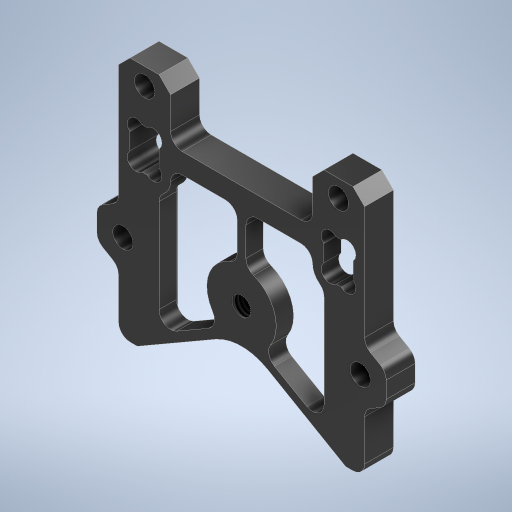
# Autodesk Inventor part: LegBaseBackFulcrumFrame
Saved by Autodesk Inventor 2024.2 (Build 282272000, 272)
## iProperties
Created: 2024-01-07
Part Number: LegBaseBackFulcrumFrame
Material: Aluminum 7075
Document SubType Name: Modeling
Designer: Masato Kubotera
Density: 2.81 g/cm^3
Appearance: Glossy - Black
Mass: 9.74355 g
Surface Area: 36.5407 cm^2
Volume: 3.46745 cm^3
Vendor: meviy
Author: Masato Kubotera
Autodesk Inventor part; units mm, degrees
ref_plane "YZ Plane" through (0, 0, 0) normal (1, 0, 0) x (0, 1, 0)
ref_plane "XZ Plane" through (0, 0, 0) normal (0, 1, 0) x (-1, 0, 0)
ref_plane "XY Plane" through (0, 0, 0) normal (0, 0, 1) x (1, 0, 0)
sketch "Sketch1" plane through (0, 0, 0) normal (1, 0, 0) x (0, 1, 0)
  line L0 (-16, 16) -> (16, 16) construction
  line L1 (16, 16) -> (16, -27) construction
  line L2 (16, -27) -> (-16, -27) construction
  line L3 (-16, -27) -> (-16, 16) construction
  line L4 (-16, 16) -> (16, -27) construction
  line L5 (16, 16) -> (-16, -27) construction
  line L6 (-13.5, 13) -> (13.5, 13) construction
  line L7 (13.5, 13) -> (13.5, -14) construction
  line L8 (13.5, -14) -> (-13.5, -14) construction
  line L9 (-13.5, -14) -> (-13.5, 13) construction
  line L10 (-13.5, 13) -> (13.5, -14) construction
  line L11 (13.5, 13) -> (-13.5, -14) construction
  line L12 (0, 18) -> (0, -27)
  circle A0 centre (0, -15) radius 8 construction
  circle A1 centre (0, 0) radius 6 construction
  line L13 (25, 27.5) -> (-25, 27.5) construction
  line L14 (19.3, 18.55) -> (14.2, 18.55)
  line L15 (14.2, 18.55) -> (14.2, 11.45)
  line L16 (14.2, 11.45) -> (19.3, 11.45)
  line L17 (19.3, 11.45) -> (19.3, 18.55)
  line L18 (19.3, 18.55) -> (14.2, 11.45) construction
  line L19 (14.2, 18.55) -> (19.3, 11.45) construction
  line L20 (-16.05, -6) -> (-16.05, 16)
  line L21 (-16.05, 16) -> (16.05, 16)
  line L22 (16.05, 16) -> (16.05, -13.8742)
  line L23 (12.25, 27.5) -> (12.25, 18)
  line L24 (12.25, 18) -> (-12.25, 18)
  line L25 (-12.25, 18) -> (-12.25, 27.5)
  arc A2 (19.3, 16.4287) -> (17.1787, 18.55) centre (18.2393, 17.4893) ccw
  line L26 (19.3, 15) -> (14.2, 15) construction
  line L27 (16.75, 18.55) -> (16.75, 11.45) construction
  arc A3 (16.3213, 18.55) -> (14.2, 16.4287) centre (15.2607, 17.4893) ccw
  arc A4 (17.1787, 11.45) -> (19.3, 13.5713) centre (18.2393, 12.5107) ccw
  arc A5 (14.2, 13.5713) -> (16.3213, 11.45) centre (15.2607, 12.5107) ccw
  line L28 (17.5, -1.7321) -> (17.5, 1.7321) construction
  line L29 (17.5, 1.7321) -> (20.5, 3.4641) construction
  line L30 (20.5, 3.4641) -> (23.5, 1.7321) construction
  line L31 (23.5, 1.7321) -> (23.5, -1.7321) construction
  line L32 (23.5, -1.7321) -> (20.5, -3.4641) construction
  line L33 (20.5, -3.4641) -> (17.5, -1.7321) construction
  line L34 (-25, 5) -> (19.25, 5) construction
  circle A6 centre (20.5, 0) radius 2.75 construction
  line L35 (16.05, 0) -> (25, 0) construction
  line L36 (20.5, 3.5218) -> (23.55, 1.7609)
  line L37 (23.55, 1.7609) -> (23.55, -1.7609)
  line L38 (23.55, -1.7609) -> (20.5, -3.5218)
  line L39 (20.5, -3.5218) -> (17.45, -1.7609)
  line L40 (17.45, -1.7609) -> (17.45, 1.7609)
  line L41 (17.45, 1.7609) -> (20.5, 3.5218)
  arc A7 (21.799, 2.7718) -> (19.201, 2.7718) centre (20.5, 2.0218) ccw
  arc A8 (18.749, 2.5109) -> (17.45, 0.2609) centre (18.749, 1.0109) ccw
  arc A9 (17.45, -0.2609) -> (18.749, -2.5109) centre (18.749, -1.0109) ccw
  arc A10 (19.201, -2.7718) -> (21.799, -2.7718) centre (20.5, -2.0218) ccw
  arc A11 (22.251, -2.5109) -> (23.55, -0.2609) centre (22.251, -1.0109) ccw
  arc A12 (23.55, 0.2609) -> (22.251, 2.5109) centre (22.251, 1.0109) ccw
  line L42 (21.25, 27.5) -> (21.25, 4.7631)
  line L43 (21.25, 4.7631) -> (25, 2.5981)
  line L44 (4.5, -7.2058) -> (18, -15)
  line L45 (21.25, -4.7631) -> (25, -2.5981)
  line L46 (21.25, -4.7631) -> (21.25, -15)
  arc A13 (4.5, -7.2058) -> (0, -6) centre (0, -15) ccw
  line L47 (19.25, 18.5) -> (14.25, 18.5) construction
  line L48 (14.25, 18.5) -> (14.25, 11.5) construction
  line L49 (14.25, 11.5) -> (19.25, 11.5) construction
  line L50 (19.25, 11.5) -> (19.25, 18.5) construction
  line L51 (19.25, 18.5) -> (14.25, 11.5) construction
  line L52 (14.25, 18.5) -> (19.25, 11.5) construction
  arc A14 (5.25, -5.9067) -> (3.2786, -5.025) centre (0, -15) ccw
  line L53 (5.25, -5.9067) -> (14.25, -11.1029)
  line L54 (14.25, -11.1029) -> (14.25, 9.686)
  line L55 (0, 0) -> (25, 0) construction
  line L56 (0.75, 14.5) -> (12.7, 14.5)
  line L57 (12.7, 14.5) -> (12.7, 14.0737)
  arc A15 (12.7, 14.0737) -> (14.25, 9.686) centre (15.2607, 12.5107) ccw
  arc A16 (3.2786, -5.025) -> (0.75, 5.9529) centre (0, 0) ccw
  line L58 (0.75, 14.5) -> (0.75, 5.9529)
  line L59 (25, 2.5981) -> (25, -2.5981)
  line L60 (21.25, 27.5) -> (12.25, 27.5)
  line L61 (18, -15) -> (21.25, -15)
  point P0 (0, -5.5)
  point P1 (0, -0.5)
  point P2 (16.05, -6)
  point P3 (16.3213, 11.45)
  point P4 (14.2, 13.5713)
  point P5 (14.2, 16.4287)
  point P6 (16.3213, 18.55)
  point P7 (19.3, 13.5713)
  point P8 (17.1787, 11.45)
  point P9 (17.45, 1.7609)
  point P10 (17.45, -1.7609)
  point P11 (20.5, -3.5218)
  point P12 (23.55, -1.7609)
  point P13 (23.55, 1.7609)
  point P14 (17.45, 0.2609)
  point P15 (17.45, -0.2609)
  point P16 (18.749, -2.5109)
  point P17 (19.201, -2.7718)
  point P18 (21.799, -2.7718)
  point P19 (22.251, -2.5109)
  point P20 (23.55, -0.2609)
  point P21 (23.55, 0.2609)
  point P22 (22.251, 2.5109)
  point P23 (18.749, 2.5109)
  point P24 (16.75, 24.5)
  point P25 (16.75, 15)
  point P26 (16.75, 15)
  point P27 (16.05, 11.2351)
  point P28 (14.2, 16)
  point P29 (0, 16)
  point P30 (5.9529, -0.75)
  dimension "d0" = 32
  dimension "d1" = 43
  dimension "d2" = 27
  dimension "d4" = 16
  dimension "d5" = 15
  dimension "d12" = 8.5
  dimension "d13" = 9.5
  dimension "d72" = 12
  dimension "d75" = 27.5
  dimension "d83" = 2
  dimension "d84" = 1.5
  dimension "d86" = 6
  dimension "d89" = 5
  dimension "d90" = 5.5
  dimension "d91" = 0.05
  dimension "d94" = 360
  dimension "d104" = 3
  dimension "d110" = 60
  dimension "d111" = 0.05
  dimension "d112" = 0.05
  dimension "d113" = 9
  dimension "d114" = 6.5
  dimension "d115" = 28.5
  dimension "d116" = 2
  dimension "d117" = 5
  dimension "d118" = 0.05
  dimension "d120" = 1.5
  dimension "d124" = 1.5
  dimension "d127" = 1.5
  dimension "d129" = 1.5
  dimension "d130" = 1.5
  dimension "d131" = 1.5
  dimension "d132" = 1.5
  dimension "d134" = 1.5
  dimension "d135" = 27
  constraints: 125 end point, 32 point on circle, 18 point on line, 17 centre point, 15 midpoint, 11 symmetric about line, 9 horizontal, 8 coincident, 8 parallel, 8 vertical, 4 collinear, 4 perpendicular, 3 tangent, 1 equal radius, 63 other
  measures "d0" distance of L1.end L2.end
  measures "d1" distance of L0.end L1.end
  measures "d2" distance of L7.end L8.end
  measures "d4" diameter of A0
  measures "d5" distance of A0.centre point (0, 0)
  measures "d12" distance from line of point (0, -5.5) L8
  measures "d13" distance of A0.centre point (0, -5.5)
  measures "d72" diameter of A1
  measures "d75" distance from line of L13 point (0, 0)
  measures "d83" distance between parallel lines of L21 L24
  measures "d84" radius of A2
  measures "d86" distance between parallel lines of L28 L31
  measures "d89" distance from line of point (0, 0) L34
  measures "d90" diameter of A6
  measures "d91" distance between parallel lines of L29 L41
  measures "d104" distance from line of L13 point (16.75, 24.5)
  measures "d110" angle of L12 L44
  measures "d111" distance between parallel lines of L50 L17
  measures "d112" distance between parallel lines of L47 L14
  measures "d113" distance between parallel lines of L47 L13
  measures "d114" distance between parallel lines of L34 L49
  measures "d115" diameter of L48 L12
  measures "d116" distance between parallel lines of L48 L23
  measures "d117" distance between parallel lines of L50 L48
  measures "d118" distance between parallel lines of L1 L22
  measures "d120" distance between parallel lines of L44 L53
  measures "d124" distance between parallel lines of L56 L21
  measures "d127" radial gap between concentric circles of A15 A5
  measures "d129" distance between parallel lines of L15 L57
  measures "d130" diameter of L58 L12
  measures "d131" distance between parallel lines of L28 L1
  measures "d132" distance between parallel lines of L30 L43
  measures "d134" distance between parallel lines of L59 L31
  measures "d135" distance between parallel lines of L8 L6
extrude "Extrusion1" add sketch "Sketch1" along normal blind 5 contours L24 L23 L60 L42 L43 L59 L45 L46 L61 L44 L22 A5 L16 A4 L17 A2 L14 A3 L15 L21 L12 | L21 L15 A5 L22 L44 A13 L12 | A7 L36 | L36 L37 L38 L39 L40 L41 | L41 A7 | A12 L36 | L41 A8 | A12 L37 | L40 A8 | A11 L37 | L40 A9 | A11 L38 | L39 A9 | A10 L38 | L39 A10
extrude "Extrusion2" cut sketch "Sketch1" along normal blind 2 contours L21 L15 A5 L22 L44 A13 L12 | A7 L36 | L36 L37 L38 L39 L40 L41 | L41 A7 | A12 L36 | L41 A8 | A12 L37 | L40 A8 | A11 L37 | L40 A9 | A11 L38 | L39 A9 | A10 L38 | L39 A10 | A14 A16 L58 L56 L57 A15 L54 L53
hole "M4" at (0, 0, 0) direction (1, 0, 0) diameter 3.242 end through all thread size "M4x0.7" class "6H" standard "ANSI Metric M Profile"
hole "Phi3.5" at (0, 20.5, 0) at (0, 16.75, 24.5) direction (1, 0, 0) diameter 3.5 end through all
fillet "R2" radius 2 13 edges at (2.5, 12.25, 18) (2.5, 21.25, -4.7631) (2.5, 21.25, -15) (3.5, 14.25, -11.1029) (3.5, 3.2786, -5.025) (3.5, 12.7, 14.5) (3.5, 12.7, 14.0737) (3.5, 0.75, 5.9529) (3.5, 0.75, 14.5) (2.5, 21.25, 4.7631) (2.5, 25, 2.5981) (2.5, 25, -2.5981) (3.5, 14.25, 9.686)
chamfer "C2" distance 2 angle 45 2 edges at (2.5, 12.25, 27.5) (2.5, 21.25, 27.5)
mirror "Mirror1" about plane through (0, 0, 0) normal (0, 1, 0)
body "Solid1"
